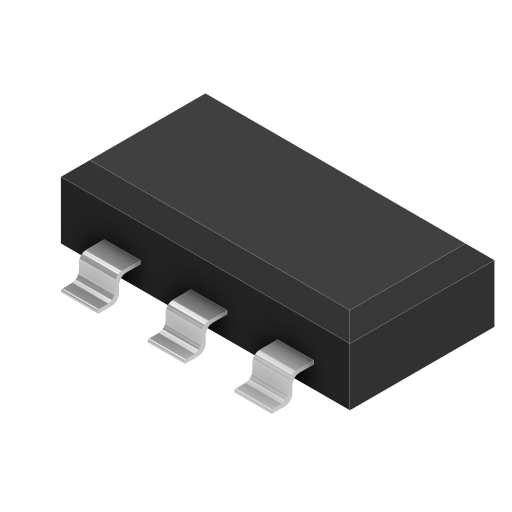
# Autodesk Inventor part: 3V DC Regulator
Saved by Autodesk Inventor 2024 (Build 280153000, 153)
## iProperties
Created: 2024-09-24
Part Number: 3V DC Regulator
Material: Generic
Document SubType Name: Modeling
Designer: Laith Al-Sadi
Density: 1 g/cm^3
Appearance: Rubber - Black
Author: Laith Al-Sadi
Autodesk Inventor part; units mm, degrees
ref_plane "YZ Plane" through (0, 0, 0) normal (1, 0, 0) x (0, 1, 0)
ref_plane "XZ Plane" through (0, 0, 0) normal (0, 1, 0) x (-1, 0, 0)
sketch "Sketch1" plane through (0, 0, 0) normal (0, 1, 0) x (-1, 0, 0)
  line L0 (2, 1) -> (-2, 1)
  line L1 (-2, 1) -> (-2, -1)
  line L2 (-2, -1) -> (2, -1)
  line L3 (2, -1) -> (2, 1)
  line L4 (2, 1) -> (-2, -1) construction
  line L5 (-2, 1) -> (2, -1) construction
  point P0 (0, 0)
  dimension "d0" = 4
  dimension "d1" = 2
  constraints: 12 end point, 2 midpoint, 2 parallel, 1 horizontal, 1 perpendicular
  measures "d0" distance of L1.end L2.end
  measures "d1" distance of L2.end L0.start
extrude "Extrusion1" add sketch "Sketch1" along normal blind 1
chamfer "Chamfer1" distance 0.2 angle 45 4 edges at (0, 1, 1) (2, 1, 0) (0, 1, -1) (-2, 1, 0)
ref_plane "Work Plane1" through (1.5, 0, 1) normal (1, 0, 0) x (0, 0, -1)
sketch "Sketch2" plane through (1.5, 0, 1) normal (1, 0, 0) x (0, 0, -1)
  line L0 (0, 0) -> (0, 0.8) projected
  line L1 (0, 0.3) -> (-0.2, 0.3)
  line L2 (-0.3, 0.2) -> (-0.3, 0.1)
  line L3 (-0.4, 0) -> (-0.575, 0)
  line L4 (0, 0) -> (2, 0) projected
  line L5 (0, 0.35) -> (-0.25, 0.35)
  line L6 (-0.35, 0.25) -> (-0.35, 0.15)
  line L7 (-0.45, 0.05) -> (-0.575, 0.05)
  line L8 (-0.6, 0.025) -> (-0.6, 0.025)
  arc A0 (-0.25, 0.35) -> (-0.35, 0.25) centre (-0.25, 0.25) ccw
  arc A1 (-0.2, 0.3) -> (-0.3, 0.2) centre (-0.2, 0.2) ccw
  arc A2 (-0.45, 0.05) -> (-0.35, 0.15) centre (-0.45, 0.15) ccw
  arc A3 (-0.4, 0) -> (-0.3, 0.1) centre (-0.4, 0.1) ccw
  arc A4 (-0.575, 0.05) -> (-0.6, 0.025) centre (-0.575, 0.025) ccw
  arc A5 (-0.6, 0.025) -> (-0.575, 0) centre (-0.575, 0.025) ccw
  point P0 (1, 0)
  point P1 (-0.3, 0.3)
  point P2 (-0.3, 0)
  point P3 (-0.6, 0)
  point P4 (0, 0.35)
  point P5 (-0.6, 0.025)
  dimension "d8" = 0.3
  dimension "d9" = 0.3
  dimension "d10" = 0.3
  dimension "d11" = 0.05
  dimension "d12" = 0.1
  dimension "d13" = 0.025
  constraints: 14 end point, 12 point on circle, 12 tangent, 7 point on line, 6 centre point, 5 perpendicular, 4 equal radius, 1 collinear, 1 vertical, 2 other
  measures "d8" distance of L1.start point (-0.3, 0.3)
  measures "d9" distance of point (-0.3, 0.3) point (-0.3, 0)
  measures "d10" distance of point (-0.3, 0) point (-0.6, 0)
  measures "d11" distance between parallel lines of L1 L5
  measures "d12" radius of A0
  measures "d13" radius of A4
extrude "Extrusion2" add sketch "Sketch2" against normal blind 0.5
pattern_linear "Rectangular Pattern1" count 3 spacing 1.2 along (-1, 0, 0) of "Extrusion2"
body "Solid1"
